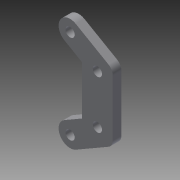
# Autodesk Inventor part: TestMount
Saved by Autodesk Inventor 2015 (Build 190159000, 159)
## iProperties
Created: 2017-03-05
Part Number: TestMount
Material: Generic
Document SubType Name: Modeling
Designer: 1esh9
Density: 1 g/cm^3
Appearance: Default
Author: 1esh9
Autodesk Inventor part; units mm, degrees
ref_plane "YZ Plane" through (0, 0, 0) normal (1, 0, 0) x (0, 1, 0)
ref_plane "XZ Plane" through (0, 0, 0) normal (0, 1, 0) x (-1, 0, 0)
ref_plane "XY Plane" through (0, 0, 0) normal (0, 0, 1) x (1, 0, 0)
sketch "Sketch1" plane through (0, 0, 0) normal (0, 1, 0) x (-1, 0, 0)
  circle A0 centre (5.65, 15.5) radius 1.6
  circle A1 centre (5.65, -15.5) radius 1.6
  arc A2 (7.65, 12.0359) -> (3.65, 18.9641) centre (5.65, 15.5) ccw
  arc A3 (3.65, -18.9641) -> (7.65, -12.0359) centre (5.65, -15.5) ccw
  line L0 (5.65, 15.5) -> (5.65, -15.5) construction
  circle A4 centre (-3.864, 8.4) radius 1.6
  circle A5 centre (-3.864, -8.4) radius 1.6
  line L1 (15.2493, 0) -> (-13.6973, 0) projected
  line L2 (0, -29.3497) -> (0, 29.3497) projected
  line L3 (-3.864, 8.4) -> (-3.864, -8.4) construction
  line L4 (-3.864, 11.8064) -> (-0.914, 10.1032)
  line L5 (-0.914, 10.1032) -> (-0.914, 6.6968)
  line L6 (-0.914, 6.6968) -> (-3.864, 4.9936)
  line L7 (-3.864, 4.9936) -> (-6.814, 6.6968)
  line L8 (-6.814, 6.6968) -> (-6.814, 10.1032)
  line L9 (-6.814, 10.1032) -> (-3.864, 11.8064)
  line L10 (-3.864, -4.9936) -> (-0.914, -6.6968)
  line L11 (-0.914, -6.6968) -> (-0.914, -10.1032)
  line L12 (-0.914, -10.1032) -> (-3.864, -11.8064)
  line L13 (-3.864, -11.8064) -> (-6.814, -10.1032)
  line L14 (-6.814, -10.1032) -> (-6.814, -6.6968)
  line L15 (-6.814, -6.6968) -> (-3.864, -4.9936)
  line L16 (-9.214, 9.805) -> (-9.214, -9.805)
  line L17 (-7.714, -12.4031) -> (3.65, -18.9641)
  line L18 (-7.714, 12.4031) -> (3.65, 18.9641)
  arc A6 (-7.714, 12.4031) -> (-9.214, 9.805) centre (-6.214, 9.805) ccw
  arc A7 (-9.214, -9.805) -> (-7.714, -12.4031) centre (-6.214, -9.805) ccw
  line L19 (7.65, 12.0359) -> (1.486, 8.4771)
  line L20 (1.486, 8.4771) -> (1.486, -8.4771)
  line L21 (1.486, -8.4771) -> (7.65, -12.0359)
  point P0 (0, 0)
  dimension "d0" = 31
  dimension "d2" = 3.2
  dimension "d3" = 3.2
  dimension "d6" = 8
  dimension "d7" = 8
  dimension "d32" = 16.8
  dimension "d33" = 15.5
  dimension "d34" = 8.4
  dimension "d35" = 5.65
  dimension "d36" = 3.864
  dimension "d37" = 3.2
  dimension "d38" = 3.2
  dimension "d39" = 5.9
  dimension "d40" = 5.9
  dimension "d41" = 2.4
  dimension "d42" = 3
  dimension "d45" = 2.4
  constraints: 40 end point, 8 centre point, 8 point on circle, 8 tangent, 4 coincident, 4 parallel, 3 vertical, 2 point on line, 1 equal radius, 26 other
  measures "d0" distance of A1.centre A0.centre
  measures "d2" diameter of A0
  measures "d3" diameter of A1
  measures "d6" diameter of A2
  measures "d7" diameter of A3
  measures "d32" distance of L3.end L3.start
  measures "d33" distance from line of L1 A0.centre
  measures "d34" distance from line of L1 L3.start
  measures "d35" distance between parallel lines of L2 L0
  measures "d36" distance between parallel lines of L2 L3
  measures "d37" diameter of A4
  measures "d38" diameter of A5
  measures "d39" distance between parallel lines of L8 L5
  measures "d40" distance between parallel lines of L14 L11
  measures "d41" distance between parallel lines of L8 L16
  measures "d42" radius of A6
  measures "d45" distance between parallel lines of L5 L20
extrude "Extrusion5" add sketch "Sketch1" along normal blind 3 contours L19 L20 L1 L2 L18 A2 | L2 L1 L16 A6 L18 | L20 L21 A3 L17 L2 L1 | L2 L17 A7 L16 L1 | L4 L5 L6 L7 L8 L9 | L10 L11 L12 L13 L14 L15
equation "\"d33\" = 0.5 * d0"
equation "\"d34\" = 0.5 * d32"
equation "\"d40\" = d39"
equation "\"d45\" = d41"
body "Solid2"
